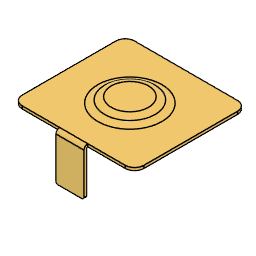
Battery+10aa (Autodesk Fusion 360 archive; units mm, degrees)
design "Battery tab +"
Autodesk Fusion 360 part; units mm, degrees
note: some values were not read from the file. Chosen so that the rebuilt part matches the saved one: a side.
sketch "Sketch1" plane through (0, 0, 0) normal (0, 1, 0) x (1, 0, 0)
  line L0 (-6.5, 6) -> (6.5, 6)
  line L1 (6.5, 6) -> (6.5, -6)
  line L2 (6.5, -6) -> (-6.5, -6)
  line L3 (-6.5, -6) -> (-6.5, 6)
  line L4 (-6.5, 6) -> (6.5, -6) construction
  line L5 (6.5, 6) -> (-6.5, -6) construction
  dimension "d1" = 13
  dimension "d2" = 12
  constraint horizontal L0
  constraint perpendicular L0 L1
  constraint parallel L0 L2
  constraint parallel L1 L3
  constraint coincident L4 origin
  constraint coincident L5 origin
  measures "d1" distance of L1.end L2.end
  measures "d2" distance of L0.end L1.end
extrude "Extrude1" add sketch "Sketch1" along normal blind 0.3
sketch "Sketch2" plane through (0, 0.3, 0) normal (0, 1, 0) x (-1, 0, 0)
  line L0 (6.5, 6) -> (-6.5, 6)
  line L1 (-6.5, 6) -> (-6.5, -6)
  line L2 (-6.5, -6) -> (6.5, -6)
  line L3 (6.5, -6) -> (6.5, 6)
  line L4 (-6.5, 0) -> (-0.5, 0) construction
  line L5 (-0.5, 0) -> (-0.5, -6) construction
  line L6 (0, -6) -> (0, 6) construction
  circle A0 centre (-0.5, 0) radius 1.5
  point P0 (-0.5, 0)
  point P1 (0.5, 0)
  dimension "d16" = 3
  constraint midpoint L1 L4.start
  constraint perpendicular L1 L4
  constraint coincident L2 L5.end
  constraint perpendicular L2 L5
  constraint midpoint L2 L6.start
  constraint midpoint L0 L6.end
  constraint coincident P0 L4.end
  constraint equal L4 L5
  constraint symmetric P0 L6 P1
  measures "d16" diameter of A0
sketch "Sketch3" plane through (0, 0.3, 0) normal (0, 1, 0) x (-1, 0, 0)
  line L0 (6.5, 6) -> (-6.5, 6)
  line L1 (-6.5, 6) -> (-6.5, -6)
  line L2 (-6.5, -6) -> (6.5, -6)
  line L3 (6.5, -6) -> (6.5, 6)
  circle A0 centre (0, 0) radius 2.5
  point P0 (0.5, 0)
  dimension "d5" = 5
  constraint coincident A0.centre origin
  measures "d5" diameter of A0
extrude "Extrude2" add sketch "Sketch3" along normal blind 0.6 contours A0
fillet "Fillet1" radius 1 2 edges at (2.3308, 0.3, 0.904) (2.3308, 0.9, -0.904)
shell "Shell1" thickness 0.3 removed faces 1 at (2.1667, 0, 2)
fillet "Fillet2" radius 1 4 edges at (-6.5, 0.15, 6) (-6.5, 0.15, -6) (6.5, 0.15, -6) (6.5, 0.15, 6)
sketch "Sketch7" plane through (0, 0, 0) normal (1, 0, 0) x (0, 0, -1)
  line L0 (-6, 0) -> (-6, 0.3)
  line L1 (-6, 0.3) -> (-6.4, 0.3)
  line L2 (-6.4, 0.3) -> (-6.4, -4.7)
  dimension "d35" = 0.4
  dimension "d36" = 5
  constraint coincident L0.end L1.start
  constraint perpendicular L0 L1
  constraint perpendicular L1 L2
  measures "d35" distance of L0.end L1.end
  measures "d36" distance of L1.end L2.end
extrude "Extrude6" add sketch "Sketch7" along normal mid plane 3 thin wall 0.3 on the left open curves L1 L2
fillet "Fillet7" radius 0.4 1 edges at (0, 0.3, 6.4)
fillet "Fillet8" radius 0.1 1 edges at (0, 0, 6.1)
fillet "Fillet9" radius 0.2 2 edges at (1.5, -4.7, 6.25) (-1.5, -4.7, 6.25)
